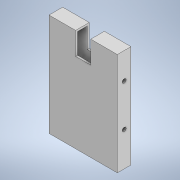
# Autodesk Inventor part: Heatsink Jig
Saved by Autodesk Inventor 2020 (Build 240168000, 168)
## iProperties
Created: 2021-03-24
Part Number: Heatsink Jig
Material: Generic
Document SubType Name: Modeling
Designer: dkiiv
Density: 1 g/cm^3
Appearance: Default
Author: dkiiv
Autodesk Inventor part; units mm, degrees
ref_plane "YZ Plane" through (0, 0, 0) normal (1, 0, 0) x (0, 1, 0)
ref_plane "XZ Plane" through (0, 0, 0) normal (0, 1, 0) x (-1, 0, 0)
ref_plane "XY Plane" through (0, 0, 0) normal (0, 0, 1) x (1, 0, 0)
sketch "Sketch1" plane through (0, 0, 0) normal (0, 0, 1) x (1, 0, 0)
  line L0 (0, 0) -> (60, 0)
  line L1 (60, 0) -> (60, 100)
  line L2 (60, 100) -> (0, 100)
  line L3 (0, 100) -> (0, 0)
  line L4 (-5, 0) -> (65, 0)
  line L5 (65, 0) -> (65, 105)
  line L6 (65, 105) -> (-5, 105)
  line L7 (-5, 105) -> (-5, 0)
  dimension "d0" = 60
  dimension "d1" = 100
  dimension "d2" = 5
  dimension "d3" = 5
  dimension "d4" = 5
  constraints: 16 end point, 4 parallel, 2 horizontal, 2 perpendicular, 1 point on line
  measures "d0" distance of L2.end L1.end
  measures "d1" distance of L1.end L0.end
  measures "d2" distance between parallel lines of L6 L2
  measures "d3" distance between parallel lines of L5 L1
  measures "d4" distance between parallel lines of L3 L7
extrude "Extrusion1" add sketch "Sketch1" along normal blind 14
sketch "Sketch2" plane through (-5, 0, 0) normal (0, -1, 0) x (1, 0, 0)
  line L0 (5, 2) -> (65, 2)
  line L1 (65, 2) -> (65, 12)
  line L2 (65, 12) -> (5, 12)
  line L3 (5, 12) -> (5, 2)
  line L4 (0, 14) -> (70, 14) projected
  line L5 (0, 0) -> (70, 0) projected
  line L6 (70, 0) -> (70, 14) projected
  line L7 (0, 0) -> (0, 14) projected
  point P0 (5, 0)
  dimension "d7" = 2
  dimension "d8" = 2
  dimension "d9" = 5
  dimension "d10" = 5
  constraints: 8 end point, 2 parallel, 1 horizontal, 1 perpendicular
  measures "d7" distance between parallel lines of L4 L2
  measures "d8" distance between parallel lines of L5 L0
  measures "d9" distance between parallel lines of L6 L1
  measures "d10" distance between parallel lines of L7 L3
extrude "Extrusion2" cut sketch "Sketch2" against normal blind 103 contours L3 L2 L1 L0
sketch "Sketch3" plane through (0, 0, 14) normal (0, 0, 1) x (1, 0, 0)
  line L0 (37.75, 103) -> (22.25, 103)
  line L1 (22.25, 103) -> (22.25, 82)
  line L2 (22.25, 82) -> (37.75, 82)
  line L3 (37.75, 82) -> (37.75, 103)
  line L4 (65, 105) -> (-5, 105) projected
  line L5 (0, 0) -> (0, 103) projected
  line L6 (0, 103) -> (60, 103) projected
  line L7 (0, 103) -> (60, 103)
  line L8 (60, 0) -> (60, 103) projected
  line L9 (22.25, 103) -> (22.25, 105)
  line L10 (65, 105) -> (-5, 105) projected
  line L11 (37.75, 103) -> (37.75, 105)
  line L12 (22.25, 105) -> (37.75, 105)
  dimension "d13" = 2
  dimension "d14" = 22.25
  dimension "d15" = 15.5
  dimension "d16" = 21
  dimension "d17" = 60
  dimension "d18" = 22.25
  constraints: 16 end point, 4 perpendicular, 3 equal length, 2 point on line, 1 horizontal
  measures "d13" distance between parallel lines of L4 L0
  measures "d14" distance between parallel lines of L1 L5
  measures "d15" distance of L1.end L2.end
  measures "d16" distance of L2.end L0.start
  measures "d17" distance of L5.end L6.end
  measures "d18" distance between parallel lines of L8 L3
extrude "Extrusion3" cut sketch "Sketch3" against normal up to surface (14 mm away)
sketch "Sketch4" plane through (65, 0, 0) normal (1, 0, 0) x (0, 0, -1)
  circle A0 centre (-7, 78) radius 2
  circle A1 centre (-7, 35) radius 2
  line L0 (-12, 103) -> (-2, 103) projected
  line L1 (-12, 0) -> (-12, 103) projected
  line L2 (0, 0) -> (-14, 0) projected
  dimension "d21" = 4
  dimension "d22" = 4
  dimension "d23" = 25
  dimension "d24" = 5
  dimension "d25" = 35
  dimension "d26" = 5
  constraints: 2 centre point
  measures "d21" diameter of A0
  measures "d22" diameter of A1
  measures "d23" distance from line of L0 A0.centre
  measures "d24" distance from line of L1 A0.centre
  measures "d25" distance from line of L2 A1.centre
  measures "d26" distance from line of L1 A1.centre
extrude "Extrusion4" cut sketch "Sketch4" against normal up to surface (42.75 mm away)
body "Solid1"
